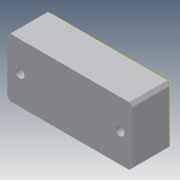
# Autodesk Inventor part: victorsp
Saved by Autodesk Inventor 2014 (Build 180170000, 170)
## iProperties
Created: 2016-01-12
Part Number: victorsp
Material: Generic
Document SubType Name: Modeling
Designer: Paul
Density: 1 g/cm^3
Appearance: Default
Author: Paul
Autodesk Inventor part; units mm, degrees
ref_plane "YZ Plane" through (0, 0, 0) normal (1, 0, 0) x (0, 1, 0)
ref_plane "XZ Plane" through (0, 0, 0) normal (0, 1, 0) x (-1, 0, 0)
ref_plane "XY Plane" through (0, 0, 0) normal (0, 0, 1) x (1, 0, 0)
sketch "Sketch1" plane through (0, 0, 0) normal (0, 0, 1) x (1, 0, 0)
  line L0 (0, 0) -> (63.5, 0)
  line L1 (63.5, 0) -> (63.5, 29.718)
  line L2 (63.5, 29.718) -> (0, 29.718)
  line L3 (0, 29.718) -> (0, 0)
  dimension "d0" = 63.5
  dimension "d1" = 29.718
  constraints: 8 end point, 2 parallel, 1 coincident, 1 horizontal, 1 perpendicular
  measures "d0" distance of L2.end L1.end
  measures "d1" distance of L1.end L0.end
extrude "Extrusion1" add sketch "Sketch1" along normal blind 20.6375
sketch "Sketch2" plane through (0, 0, 20.6375) normal (0, 0, 1) x (1, 0, 0)
  line L0 (63.5, 0) -> (63.5, 29.718) projected
  line L1 (63.5, 29.718) -> (0, 29.718) projected
  line L2 (0, 29.718) -> (0, 0) projected
  line L3 (6.35, 14.859) -> (57.15, 14.859)
  point P0 (0, 14.859)
  point P1 (63.5, 14.859)
  point P2 (31.75, 14.859)
  point P3 (31.75, 29.718)
  dimension "d4" = 50.8
  constraints: 4 midpoint, 2 end point, 2 horizontal alignment, 1 perpendicular, 1 vertical alignment
  measures "d4" distance of L3.end L3.start
hole "Hole1" at (6.35, 14.859, 20.6375) at (57.15, 14.859, 20.6375) direction (0, 0, -1) diameter 4.7625 depth 25.4 tip angle 118
chamfer "Chamfer1" distance 1.524 angle 45 8 edges at (63.5, 29.718, 10.3188) (0, 29.718, 10.3188) (63.5, 0, 10.3188) (0, 0, 10.3188) (31.75, 29.718, 0) (63.5, 14.859, 0) (31.75, 0, 0) (0, 14.859, 0)
sketch "Sketch3" plane through (0, 0, 0) normal (0, 0, -1) x (-1, 0, 0)
  circle A0 centre (-57.15, 14.859) radius 2.3813 projected
  circle A1 centre (-6.35, 14.859) radius 2.3813 projected
  line L0 (-1.524, 1.524) -> (-61.976, 1.524) projected
  line L1 (-1.524, 28.194) -> (-1.524, 1.524) projected
  line L2 (-61.976, 28.194) -> (-1.524, 28.194) projected
  line L3 (-61.976, 1.524) -> (-61.976, 28.194) projected
  line L4 (-46.4581, 22.2961) -> (-17.9931, 22.2961) construction
  line L5 (-17.9931, 22.2961) -> (-17.9931, 6.8261) construction
  line L6 (-17.9931, 6.8261) -> (-46.4581, 6.8261) construction
  line L7 (-46.4581, 6.8261) -> (-46.4581, 22.2961) construction
  point P0 (0, 0)
  constraints: 2 other
body "Solid1"
